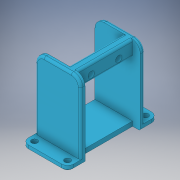
# Autodesk Inventor part: Stewart-Small-Servo-Holder
Saved by Autodesk Inventor 2018.2 (Build 222227000, 227)
## iProperties
Created: 2018-02-17
Part Number: Stewart-Small-Servo-Holder
Material: Generisch
Document SubType Name: Modeling
Designer: JochenAlt
Density: 1 g/cm^3
Appearance: Vorgabe
Author: JochenAlt
Autodesk Inventor part; units mm, degrees
ref_plane "YZ Plane" through (0, 0, 0) normal (1, 0, 0) x (0, 1, 0)
ref_plane "XZ Plane" through (0, 0, 0) normal (0, 1, 0) x (-1, 0, 0)
ref_plane "XY Plane" through (0, 0, 0) normal (0, 0, 1) x (1, 0, 0)
sketch "Skizze1" plane through (0, 0, 0) normal (0, 0, 1) x (1, 0, 0)
  line L0 (0, 28.6429) -> (0, -28.6429) construction
  line L1 (-50.7, 0) -> (8.45, 0) construction
  line L2 (-42.25, 11.9) -> (-10, 11.9) construction
  line L3 (-10, 11.9) -> (-10, -11.9) construction
  line L4 (-10, -11.9) -> (-42.25, -11.9) construction
  line L5 (-42.25, -11.9) -> (-42.25, 11.9) construction
  line L6 (-11.1, 11.9) -> (-11.1, -11.9) construction
  line L7 (-13.1, 11.9) -> (-13.1, -11.9) construction
  line L8 (-10, 0.25) -> (-42.25, 0.25) construction
  line L9 (-10, -0.25) -> (-42.25, -0.25) construction
  line L10 (-30, 14.2) -> (-30, -14.2)
  line L11 (-30, 12.2) -> (-10, 12.2)
  line L12 (-30, 14.2) -> (-10, 14.2)
  line L13 (-30, -12.2) -> (-10, -12.2)
  line L14 (-30, -14.2) -> (-10, -14.2)
  line L15 (-10, 14.2) -> (-10, -14.2)
  line L16 (-27.3, -19.9) -> (-12.7, -19.9)
  line L17 (-27.3, 19.9) -> (-12.7, 19.9)
  line L18 (-30, -14.2) -> (-30, -17.2)
  line L19 (-10, -14.2) -> (-10, -17.2)
  line L20 (-30, 14.2) -> (-30, 17.2)
  line L21 (-10, 14.2) -> (-10, 17.2)
  arc A0 (-30, -17.2) -> (-27.3, -19.9) centre (-27.3, -17.2) ccw
  arc A1 (-12.7, -19.9) -> (-10, -17.2) centre (-12.7, -17.2) ccw
  arc A2 (-10, 17.2) -> (-12.7, 19.9) centre (-12.7, 17.2) ccw
  arc A3 (-27.3, 19.9) -> (-30, 17.2) centre (-27.3, 17.2) ccw
  circle A4 centre (-27.3, -17.2) radius 1.3
  circle A5 centre (-12.7, -17.2) radius 1.3
  circle A6 centre (-27.3, 17.2) radius 1.3
  circle A7 centre (-12.7, 17.2) radius 1.3
  line L22 (-28, 9.075) -> (-26, 9.075) construction
  line L23 (-25, 8.075) -> (-25, 4.075) construction
  line L24 (-26, 3.075) -> (-28, 3.075) construction
  line L25 (-29, 4.075) -> (-29, 8.075) construction
  line L26 (-28, -3.075) -> (-26, -3.075) construction
  line L27 (-25, -4.075) -> (-25, -8.075) construction
  line L28 (-26, -9.075) -> (-28, -9.075) construction
  line L29 (-29, -8.075) -> (-29, -4.075) construction
  arc A8 (-28, 9.075) -> (-29, 8.075) centre (-28, 8.075) ccw construction
  arc A9 (-25, 8.075) -> (-26, 9.075) centre (-26, 8.075) ccw construction
  arc A10 (-26, 3.075) -> (-25, 4.075) centre (-26, 4.075) ccw construction
  arc A11 (-29, 4.075) -> (-28, 3.075) centre (-28, 4.075) ccw construction
  arc A12 (-28, -3.075) -> (-29, -4.075) centre (-28, -4.075) ccw construction
  arc A13 (-29, -8.075) -> (-28, -9.075) centre (-28, -8.075) ccw construction
  arc A14 (-26, -9.075) -> (-25, -8.075) centre (-26, -8.075) ccw construction
  arc A15 (-25, -4.075) -> (-26, -3.075) centre (-26, -4.075) ccw construction
  line L30 (-13.4, 12.2) -> (-13.4, -12.2)
  line L31 (-10.8, 12.2) -> (-10.8, -12.2)
  line L32 (-17.4, -12.2) -> (-17.4, 12.2)
  line L33 (-30, -6.075) -> (-10, -6.075) construction
  line L34 (-30, 11.9) -> (-30, -11.9) construction
  line L35 (-10, 11.9) -> (-10, -11.767) construction
  point P0 (0, 0)
  dimension "d5" = 0.5
  dimension "d10" = 32.25
  dimension "d13" = 0.3
  dimension "d40" = 11.65
  dimension "d43" = 2.7
  dimension "d46" = 10
  dimension "d47" = 2.6
  dimension "d59" = 2
  dimension "d60" = 5.7
  dimension "d61" = 2
  dimension "d63" = 1
  dimension "d64" = 6
  dimension "d65" = 4
  dimension "d67" = 0.3
  dimension "d68" = 0.3
  dimension "d69" = 4
  dimension "d76" = 16.9
  dimension "d77" = 20
  dimension "d78" = 0
  dimension "d79" = 0
  dimension "d80" = 1
  constraints: 68 end point, 24 point on circle, 24 point on line, 24 tangent, 16 centre point, 13 equal radius, 13 parallel, 10 perpendicular, 7 vertical, 5 horizontal, 4 coincident, 2 collinear, 9 other
  measures "d5" distance between parallel lines of L9 L8
  measures "d10" distance between parallel lines of L5 L3
  measures "d13" distance between parallel lines of L2 L11
  measures "d40" distance between parallel lines of L8 L2
  measures "d43" radius of A0
  measures "d46" distance between parallel lines of L0 L3
  measures "d47" diameter of A4
  measures "d59" distance between parallel lines of L11 L12
  measures "d60" distance between parallel lines of L17 L12
  measures "d61" distance between parallel lines of L6 L7
  measures "d63" radius of A8
  measures "d64" distance between parallel lines of L24 L22
  measures "d65" distance between parallel lines of L23 L25
  measures "d67" distance between parallel lines of L7 L30
  measures "d68" distance between parallel lines of L6 L31
  measures "d69" distance between parallel lines of L32 L30
  measures "d76" distance between parallel lines of L10 L7
  measures "d77" distance between parallel lines of L35 L34
  measures "d78" distance between parallel lines of L35 L15
  measures "d79" distance between parallel lines of L34 L10
  measures "d80" distance between parallel lines of L25 L34
extrude "Extrusion1" add sketch "Skizze1" along normal blind 2 contours L12 L15 L11 L10 | L20 A3 L17 A2 L21 L12 | L11 L32 L13 L10 | L13 L15 L14 L10 | L11 L30 L13 L32 | L14 L19 A1 L16 A0 L18
extrude "Extrusion2" add sketch "Skizze1" along normal blind 26.36 contours L12 L15 L11 L10 | L13 L15 L14 L10
extrude "Extrusion4" add sketch "Skizze1" along normal blind 2 from surface at 26.36 contours L12 L15 L11 L10 | L13 L15 L14 L10 | L11 L30 L13 L32
extrude "Extrusion5" add sketch "Skizze1" along normal blind 5 from surface at 28.36 contours L12 L15 L11 L10 | L13 L15 L14 L10 | L11 L30 L13 L32
sketch "Skizze4" plane through (-13.4, -12.2, 26.36) normal (1, 0, 0) x (0, 0, -1)
  line L0 (-7, 24.4) -> (-7, 0) construction
  line L1 (0, 0) -> (-7, 0) construction
  line L2 (0, 24.4) -> (0, 0) construction
  line L3 (-7, 24.4) -> (0, 24.4) construction
  line L4 (-7, 0) -> (-7, 24.4) construction
  line L5 (0, 24.4) -> (0, 0) construction
  line L6 (-7, 24.4) -> (-7, 0) construction
  line L7 (-7, 12.2) -> (0, 12.2) construction
  line L8 (-2.47, 6.125) -> (-2.47, 18.275) construction
  circle A0 centre (-2.47, 6.125) radius 1.4
  circle A1 centre (-2.47, 18.275) radius 1.4
  line L9 (0, 6.125) -> (26.318, 6.125) construction
  line L10 (27.8406, 18.275) -> (-7, 18.275) construction
  point P0 (26.36, 12.2)
  point P1 (28.36, 18.275)
  point P2 (28.36, 18.275)
  point P3 (28.36, 18.275)
  point P4 (26.36, 6.125)
  point P5 (26.36, 6.125)
  point P6 (26.36, 6.125)
  dimension "d70" = 2.47
  dimension "d71" = 2.8
  constraints: 8 end point, 5 point on line, 2 centre point, 2 coincident, 2 midpoint, 1 equal radius, 1 horizontal, 1 perpendicular, 1 other
  measures "d70" distance between parallel lines of L2 L8
  measures "d71" diameter of A0
extrude "Extrusion9" cut sketch "Skizze4" against normal up to next
fillet "Rundung4" radius 4 4 edges at (-10, -13.2, 33.36) (-30, -13.2, 33.36) (-10, 13.2, 33.36) (-30, 13.2, 33.36)
fillet "Rundung4" radius 1 10 edges at (-10, -14.2, 17.68) (-20, -14.2, 33.36) (-30, -14.2, 17.68) (-17.4, 0, 33.36) (-13.4, 0, 26.36) (-13.4, 0, 33.36) (-17.4, 0, 26.36) (-30, 14.2, 17.68) (-20, 14.2, 33.36) (-10, 14.2, 17.68)
chamfer "Fase2" distance 0.5 angle 45 9 edges at (-10, -14.7, 0) (-10.7908, -19.1092, 0) (-20, -19.9, 0) (-29.2092, -19.1092, 0) (-30, 0, 0) (-29.2092, 19.1092, 0) (-20, 19.9, 0) (-10.7908, 19.1092, 0) (-10, 14.7, 0)
